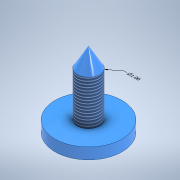
# Autodesk Inventor part: handle
Saved by Autodesk Inventor 2021.1 (Build 251245000, 245)
## iProperties
Created: 2020-08-16
Part Number: handle
Material: Generic
Document SubType Name: Modeling
Designer: robst
Density: 1 g/cm^3
Appearance: Cyan
Author: robst
Autodesk Inventor part; units mm, degrees
ref_plane "YZ Plane" through (0, 0, 0) normal (1, 0, 0) x (0, 1, 0)
ref_plane "XZ Plane" through (0, 0, 0) normal (0, 1, 0) x (-1, 0, 0)
ref_plane "XY Plane" through (0, 0, 0) normal (0, 0, 1) x (1, 0, 0)
sketch "Sketch1" plane through (0, 0, 0) normal (0, 0, 1) x (1, 0, 0)
  line L0 (0, 85.497) -> (-12.7, 63.5)
  line L1 (-12.7, 63.5) -> (-12.7, 12.7)
  line L2 (-12.7, 12.7) -> (-38.1, 12.7)
  line L3 (-38.1, 12.7) -> (-38.1, 0)
  line L4 (-38.1, 0) -> (0, 0)
  line L5 (0, 85.497) -> (0, 0)
  dimension "d1" = 0
  dimension "d2" = 12.7
  dimension "d5" = 30
  dimension "d7" = 12.7
  dimension "d14" = 50.8
  constraints: 12 end point, 3 perpendicular, 2 vertical
  measures "d1" distance of L4.end point (0, 0)
  measures "d2" vertical distance of L2.end point (0, 0)
  measures "d5" angle of L0 L5
  measures "d7" distance between parallel lines of L5 L1
  measures "d14" distance of L0.end L1.end
revolve "Revolution1" add sketch "Sketch1" angle 360 about axis through (0, 85.497, 0) along (0, -1, 0)
thread "Thread1" size "1-8 UNC" class "2A" standard "ANSI Unified Screw Threads" full length
body "Solid1"
